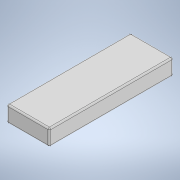
# Autodesk Inventor part: 202200606_知能ロボットanker
Saved by Autodesk Inventor 2020 (Build 240168000, 168)
## iProperties
Created: 2022-06-06
Part Number: 202200606_知能ロボットanker
Material: 一般
Document SubType Name: Modeling
Designer: Naggy
Density: 1 g/cm^3
Appearance: 既定
Author: Naggy
Autodesk Inventor part; units mm, degrees
ref_plane "YZ Plane" through (0, 0, 0) normal (1, 0, 0) x (0, 1, 0)
ref_plane "XZ Plane" through (0, 0, 0) normal (0, 1, 0) x (-1, 0, 0)
ref_plane "XY Plane" through (0, 0, 0) normal (0, 0, 1) x (1, 0, 0)
sketch "スケッチ1" plane through (0, 0, 0) normal (0, 0, 1) x (1, 0, 0)
  line L0 (-29, -11) -> (29, -11)
  line L1 (29, -11) -> (29, 11)
  line L2 (29, 11) -> (-29, 11)
  line L3 (-29, 11) -> (-29, -11)
  line L4 (-29, -11) -> (29, 11) construction
  line L5 (29, -11) -> (-29, 11) construction
  point P0 (0, 0)
  dimension "d0" = 22
  dimension "d1" = 58
  constraints: 12 end point, 2 midpoint, 2 parallel, 1 horizontal, 1 perpendicular
  measures "d0" distance between parallel lines of L0 L2
  measures "d1" distance between parallel lines of L3 L1
extrude "押し出し1" add sketch "スケッチ1" along normal blind 168
fillet "フィレット1" radius 2 12 edges at (29, 11, 84) (-29, 11, 84) (0, 11, 168) (0, -11, 168) (29, 0, 168) (-29, 0, 168) (29, -11, 84) (29, 0, 0) (0, 11, 0) (-29, 0, 0) (0, -11, 0) (-29, -11, 84)
